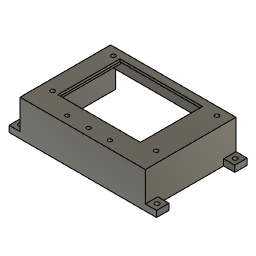
LcdMount (Autodesk Fusion 360 design; units mm, degrees)
Autodesk Fusion 360 part; units mm, degrees
sketch "screen1" plane through (0, 0, 0) normal (0, 0, 1) x (1, 0, 0)
  line L0 (-57.5, -57.0609) -> (-57.5, 0)
  line L1 (-48, -3) -> (18.5087, -3)
  line L2 (-48, -53) -> (18.5, -53)
  line L3 (-48, -3) -> (-48, -53.0003)
  circle A0 centre (30.75, -52.5) radius 1.65
  line L4 (-52.75, -52.5) -> (-52.75, -3.5) construction
  line L5 (-50.5, 0) -> (-50.5, -57.06)
  circle A1 centre (30.75, -3.5) radius 1.65
  line L6 (30.75, -52.5) -> (-52.75, -52.5) construction
  line L7 (30.75, -3.5) -> (30.75, -52.5) construction
  line L8 (-52.75, -3.5) -> (30.75, -3.5) construction
  circle A2 centre (-52.75, -52.5) radius 1.65
  circle A3 centre (-52.75, -3.5) radius 1.65
  line L9 (-61.5, -70) -> (-61.5, 3)
  line L10 (39.5, 3) -> (39.5, -70)
  line L11 (-61.5, 3) -> (39.5, 3)
  line L12 (39.5, -70) -> (-61.5, -70)
  line L13 (28.5, -48) -> (32.5, -48)
  line L14 (32.5, -8.1885) -> (28.5, -8.1885)
  line L15 (32.5, -8.1885) -> (35.5, -8.1885)
  line L16 (32.5, -48) -> (35.5, -48)
  line L17 (28.5, -57) -> (35.5, -57)
  line L18 (2.15, -61.2) -> (7.45, -61.2)
  line L19 (7.45, -61.2) -> (7.45, -66.5)
  line L20 (7.45, -66.5) -> (2.15, -66.5)
  circle A4 centre (4.8, -63.85) radius 1.5
  line L21 (2.15, -66.5) -> (2.15, -61.2)
  line L22 (-15, -61.2) -> (-9.7, -61.2)
  line L23 (-9.7, -61.2) -> (-9.7, -66.5)
  line L24 (-9.7, -66.5) -> (-15, -66.5)
  circle A5 centre (-12.35, -63.85) radius 1.5
  line L25 (-15, -66.5) -> (-15, -61.2)
  line L26 (-32.25, -61.2) -> (-26.95, -61.2)
  line L27 (-26.95, -61.2) -> (-26.95, -66.5)
  line L28 (-26.95, -66.5) -> (-32.25, -66.5)
  circle A6 centre (-29.6, -63.85) radius 1.5
  line L29 (-32.25, -66.5) -> (-32.25, -61.2)
  line L30 (-48, -68.5) -> (10, -68.5)
  line L31 (10, -59) -> (-48, -59)
  circle A7 centre (-44, -64) radius 0.9
  circle A8 centre (32, -64) radius 0.9
  line L32 (18.5, -53) -> (18.5087, -3)
  line L33 (28.5, -48) -> (28.5, -57)
  line L34 (28.5, -8.1885) -> (28.5, 0)
  line L35 (35.5, -57) -> (35.5, -48)
  line L36 (35.5, -8.1885) -> (35.5, 0)
  line L37 (-57.5, 0) -> (-50.5, 0)
  line L38 (35.5, 0) -> (28.5, 0)
  line L39 (-57.5, -57.0609) -> (-50.5, -57.06)
  line L40 (-48, -68.5) -> (-48, -59)
  line L41 (10, -68.5) -> (10, -59)
  line L42 (28.5, -68.5) -> (35.4221, -68.5)
  line L43 (35.4221, -68.5) -> (35.4221, -59)
  line L44 (35.4221, -59) -> (28.5, -59)
  line L45 (28.5, -59) -> (28.5, -68.5)
  line L46 (-48, -68.5) -> (-40, -68.5)
  line L47 (-40, -68.5) -> (-40, -59)
  line L48 (-40, -59) -> (-48, -59)
  line L49 (-48, -59) -> (-48, -68.5)
  line L50 (10, -68.5) -> (28.5, -68.5)
  line L51 (10, -59) -> (28.5, -59)
  circle A9 centre (-66, -65) radius 1.75
  circle A10 centre (-66, -65) radius 3 construction
  circle A11 centre (-66, -2) radius 1.75
  circle A12 centre (44, -65) radius 1.75
  circle A13 centre (44, -2) radius 1.75
  line L52 (-70.3285, -70) -> (-61.5, -70)
  line L53 (-61.5, -70) -> (-61.5, -60)
  line L54 (-61.5, -60) -> (-70.3285, -60)
  line L55 (-70.3285, -60) -> (-70.3285, -70)
  line L56 (39.5, -70) -> (48.5, -70)
  line L57 (48.5, -70) -> (48.5, -60)
  line L58 (48.5, -60) -> (39.5, -60)
  line L59 (39.5, -60) -> (39.5, -70)
  line L60 (-61.5, 3) -> (-70.5, 3)
  line L61 (-70.5, 3) -> (-70.5, -7)
  line L62 (-70.5, -7) -> (-61.5, -7)
  line L63 (-61.5, -7) -> (-61.5, 3)
  line L64 (39.5, 3) -> (48.5, 3)
  line L65 (48.5, 3) -> (48.5, -7)
  line L66 (48.5, -7) -> (39.5, -7)
  line L67 (39.5, -7) -> (39.5, 3)
  line L68 (-57.5, 0) -> (-57.5, 3)
  line L69 (-57.5, -57.0609) -> (-57.4986, -68.3465)
  line L70 (-57.4986, -68.3465) -> (-48, -68.5)
  line L71 (35.4221, -59) -> (35.4221, 3)
  line L72 (-57.5, 0) -> (35.5, 0)
  dimension "d24" = 83.5
  dimension "d25" = 49
  dimension "d26" = 3.3
  dimension "d27" = 3.3
  dimension "d28" = 3.3
  dimension "d29" = 3.3
  dimension "d165" = 1.8
  dimension "d166" = 1.8
  dimension "d175" = 3.5
  dimension "d176" = 6
  dimension "d177" = 3.5
  dimension "d178" = 3.5
  dimension "d179" = 3.5
  dimension "d180" = 10
  dimension "d181" = 9
  dimension "d182" = 10
  dimension "d183" = 9
  dimension "d184" = 10
  dimension "d185" = 9
  dimension "d186" = 10
  constraint vertical L0
  constraint perpendicular L2 L3
  constraint horizontal L8
  constraint vertical L7
  constraint horizontal L6
  constraint vertical L4
  constraint coincident L4.end L8.start
  constraint coincident A1.centre L7.start
  constraint coincident A0.centre L6.start
  constraint coincident L4.start L6.end
  constraint horizontal L11
  constraint vertical L10
  constraint horizontal L12
  constraint vertical L9
  constraint perpendicular L17 L33
  constraint perpendicular L16 L35
  constraint perpendicular L34 L38
  constraint perpendicular L31 L41
  constraint horizontal L42
  constraint vertical L43
  constraint horizontal L44
  constraint vertical L45
  constraint horizontal L46
  constraint vertical L47
  constraint horizontal L48
  constraint vertical L49
  constraint coincident L31 L47.end
  constraint perpendicular L45 L50
  constraint perpendicular L45 L51
  constraint concentric A9 A10
  constraint horizontal L52
  constraint vertical L53
  constraint horizontal L54
  constraint vertical L55
  constraint horizontal L56
  constraint vertical L57
  constraint horizontal L58
  constraint vertical L59
  constraint horizontal L60
  constraint vertical L61
  constraint horizontal L62
  constraint vertical L63
  constraint horizontal L64
  constraint vertical L65
  constraint horizontal L66
  constraint vertical L67
  constraint coincident L11 L68.end
  constraint perpendicular L11 L68
  constraint perpendicular L39 L69
  constraint coincident L11 L71.end
  constraint perpendicular L11 L71
  constraint perpendicular L36 L72
  measures "d24" distance of L4.end A1.centre
  measures "d25" distance of L4.end L4.start
  measures "d26" diameter of A3
  measures "d27" diameter of A1
  measures "d28" diameter of A0
  measures "d29" diameter of A2
  measures "d165" diameter of A7
  measures "d166" diameter of A8
  measures "d175" diameter of A9
  measures "d176" diameter of A10
  measures "d177" diameter of A11
  measures "d178" diameter of A12
  measures "d179" diameter of A13
  measures "d180" distance of L52.start L54.end
  measures "d181" distance of L10.end L56.end
  measures "d182" distance of L10.end L58.end
  measures "d183" distance of L9.end L60.end
  measures "d184" distance of L9.end L62.end
  measures "d185" distance of L10.start L64.end
  measures "d186" distance of L10.start L66.end
extrude "Extrude2" add sketch "screen1" along normal blind 2 contours L0 L9 L10 L11 L12 L15 L16 L17 L30 L35 L36 L38 L42 L43 L46 L50 L53 L59 L63 L67 L68 L69 L70 L71 L72 | L0 L5 L37 L39 L72 | L5 L13 L14 L15 L16 L17 L31 L33 L34 L39 L40 L44 L48 L49 L51 L69 L70 L71 L72 | L11 L37 L38 L68 L71 L72 | L30 L31 L40 L46 L47 L48 L49 | L14 L15 L34 L38 L71 L72 | L30 L31 L41 L47 | L15 L36 L38 L71 L72 | L41 L45 L50 L51 | L42 L43 L44 L45 | L13 L16 L17 L33 L71 | L16 L17 L35 L71 | L18 L19 L20 L21 | L22 L23 L24 L25 | L26 L27 L28 L29 | A7 | A8 makes body 1
extrude "Extrude4" add sketch "screen1" against normal blind 4.2 contours L0 L5 L37 L39 L72 | L14 L15 L34 L38 L71 L72 | L15 L36 L38 L71 L72 | L13 L16 L17 L33 L71 | L16 L17 L35 L71 bodies 1
extrude "Extrude38" add sketch "screen1" against normal blind 2.5 contours L30 L31 L40 L46 L47 L48 L49 | L30 L31 L41 L47 | L42 L43 L44 L45 bodies 1
extrude "Extrude39" add sketch "screen1" against normal blind 27 contours L0 L9 L10 L11 L12 L15 L16 L17 L30 L35 L36 L38 L42 L43 L46 L50 L53 L59 L63 L67 L68 L69 L70 L71 L72 bodies 1
extrude "Extrude40" add sketch "screen1" along normal blind -22 and the other way blind 27 contours L9 L60 L61 L62 L63 | L10 L64 L65 L66 L67 | L9 L52 L53 L54 L55 | L10 L56 L57 L58 L59 bodies 1
extrude "Extrude41" add sketch "screen1" against normal blind 10 contours L11 L37 L38 L68 L71 L72 bodies 1
extrude "Extrude42" add sketch "screen1" along normal blind 2 separate body contours L30 L31 L40 L46 L47 L48 L49 | L30 L31 L41 L47 | L41 L45 L50 L51 | L42 L43 L44 L45 | L18 L19 L20 L21 | A4 | L22 L23 L24 L25 | A5 | L26 L27 L28 L29 | A6 makes body 2
move_body "Move3" bodies 2 to x (1, 0, 0) y (0, 1, 0) z (0, 0, 1) at (0, 0, -5)
move_face "OffsetFaces3" offset -0.5 6 faces at (35.4221, -65.3333, -4.3333) (-45.3333, -68.5, -4.3333) (-23.3333, -68.5, -4.3333) (16.1667, -68.5, -3.6667) (30.8074, -68.5, -4.3333) (-48, -65.3333, -4.3333) on bodies 2
named bodies: "lcd_mount", "led_back_piece"
